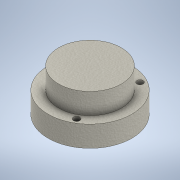
# Autodesk Inventor part: Rueda_Soporte
Saved by Autodesk Inventor 2022.1 (Build 261234000, 234)
## iProperties
Created: 2021-09-10
Part Number: Rueda_Soporte
Material: Genérico
Document SubType Name: Modeling
Designer: seb_0
Density: 1 g/cm^3
Appearance: Acero - Fundido
Author: seb_0
Autodesk Inventor part; units mm, degrees
ref_plane "YZ Plane" through (0, 0, 0) normal (1, 0, 0) x (0, 1, 0)
ref_plane "XZ Plane" through (0, 0, 0) normal (0, 1, 0) x (-1, 0, 0)
ref_plane "XY Plane" through (0, 0, 0) normal (0, 0, 1) x (1, 0, 0)
sketch "Boceto1" plane through (0, 0, 0) normal (0, 1, 0) x (-1, 0, 0)
  circle A0 centre (0, 0) radius 12.5
  circle A1 centre (0, 0) radius 20
  circle A2 centre (17.5, 0) radius 1.5
  circle A3 centre (-8.75, -15.1554) radius 1.5
  circle A4 centre (-8.75, 15.1554) radius 1.5
  line L0 (17.5, 0) -> (0, 0)
  line L1 (0, 0) -> (-8.75, -15.1554)
  line L2 (0, 0) -> (-8.75, 15.1554)
  dimension "d4" = 25
  dimension "d5" = 40
  dimension "d6" = 3
  dimension "d7" = 3
  dimension "d8" = 3
  dimension "d10" = 120
  dimension "d11" = 120
  dimension "d12" = 17.5
  dimension "d13" = 17.5
  dimension "d14" = 17.5
  constraints: 6 end point, 5 centre point, 2 coincident, 1 horizontal
  measures "d4" diameter of A0
  measures "d5" diameter of A1
  measures "d6" diameter of A2
  measures "d7" diameter of A3
  measures "d8" diameter of A4
  measures "d10" angle of L1 L2
  measures "d11" angle of L0 L2
  measures "d12" distance of L0.end L2.end
  measures "d13" distance of L0.end L1.end
  measures "d14" distance of L0.start L0.end
extrude "Extrusión1" add sketch "Boceto1" along normal blind 10
sketch "Boceto2" plane through (0, 10, 0) normal (0, 1, 0) x (1, 0, 0)
  circle A0 centre (0, 0) radius 12.5 projected
  circle A1 centre (0, 0) radius 15
  dimension "d17" = 30
  constraints: 1 centre point, 1 coincident
  measures "d17" diameter of A1
extrude "Extrusión2" add sketch "Boceto2" along normal blind 8.5
sketch "Boceto3" plane through (0, 18.5, 0) normal (0, 1, 0) x (1, 0, 0)
  circle A0 centre (0, 0) radius 15 projected
extrude "Extrusión3" add sketch "Boceto3" along normal blind 1.5
